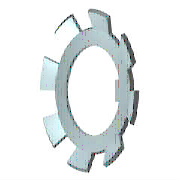
# Autodesk Inventor part: CSN 02 3640 - MB 33
Saved by Autodesk Inventor 2021 (Build 250183000, 183)
## iProperties
Created: 2020-01-21
Part Number: CSN 02 3640 - MB 33
Material: Steel, Mild
Description: Rolling bearings. Circular slotted nuts fo adapter and withdrawal sleeves
Document SubType Name: Modeling
Standard: CSN 02 3640
Designer: Angelos
Standards Organization: CSN
Language: en-US
Size Designation: MB 33
Categories: <MemberInstance><Categories><Category DisplayName="Shaft Parts" InternalName="7f7aeb1f-a693-4053-b835-cee3144e0d98" Mnemonic="SHFT"><Category DisplayName="Thrust Washers" InternalName="196297a3-bbf2-4c62-a426-6f1b43e49a92" Mnemonic="STWRDBRCMP"><CategoryParameter DisplayName="Diameter of Contact Area" InternalName="2e92645a-023d-4b6f-85cb-aa6579b07711" Mnemonic="conarea"/><CategoryParameter DisplayName="Groove Height" InternalName="459e1daf-c3a8-40cb-aa85-2a4675385d1b" Mnemonic="grvheig"/><CategoryParameter DisplayName="Thickness" InternalName="5f8ad5cd-5310-44ac-8ee3-8a10cbe3cc2a" Mnemonic="thick"/><CategoryParameter DisplayName="Shaft Diameter" InternalName="a5cdae98-95ea-47ec-9880-d704d388e74c" Mnemonic="shaftdia"/></Category></Category><Category DisplayName="DataType" InternalName="23b78d0f-2648-40c6-8793-ca6db495c9e8" Mnemonic="DATATYPE"><CategoryParameter DisplayName="DisplayName" InternalName="05415f3d-3907-474b-a020-eb9d644f4cf3" Mnemonic="DISPLAYNAME"/><CategoryParameter DisplayName="Standard" InternalName="0c0a119c-1e12-4c84-803f-101930972f5e" Mnemonic="STANDARD"/><CategoryParameter DisplayName="Description" InternalName="13903e3d-64b1-4950-80da-f627842ea37f" Mnemonic="DESCRIPTION"/><CategoryParameter DisplayName="Designation" InternalName="2675968c-4ce5-49e0-a4f5-552d29089031" Mnemonic="DESIGNATION"/><CategoryParameter DisplayName="Default Row" InternalName="2af9ec52-faaa-4026-b378-f9fa4afca842" Mnemonic="DEFAULTROW"/><CategoryParameter DisplayName="Folder Name" InternalName="3f06958e-8713-4116-9be7-ed6184ecc97b" Mnemonic="FOLDERNAME"/><CategoryParameter DisplayName="Revision Guid" InternalName="45a75005-10b1-4dfc-8d6d-dfe629f0b93c" Mnemonic="REVISIONGUID"/><CategoryParameter DisplayName="FileName" InternalName="8b46a4cc-9585-4fed-90c3-899f57e09a73" Mnemonic="FILENAME"/><CategoryParameter DisplayName="StdsOrg" InternalName="8f5914e1-4693-403f-8ab5-d37768198c9d" Mnemonic="STDSORG"/><CategoryParameter DisplayName="Family Version" InternalName="914462f6-6e19-4b14-ba84-155b9680b1d0" Mnemonic="FAMILYREVISION"/><CategoryParameter DisplayName="Standard Revision" InternalName="91d5a463-65c2-4fde-b823-3b7fea5e8e17" Mnemonic="STANDARDREVISION"/><CategoryParameter DisplayName="Member Revision" InternalName="a65d44b9-392f-4f4f-857b-e4b3d54996fe" Mnemonic="MEMBERREVISION"/><CategoryParameter DisplayName="ClipFormat" InternalName="bc51e27b-3422-4e78-93ef-cec197ddf230" Mnemonic="CLIPFORMAT"/><CategoryParameter DisplayName="Manufacturer" InternalName="cd6c7a72-a28a-4e50-99a9-2c7f4e13e5ad" Mnemonic="MANUFACTURER"/><CategoryParameter DisplayName="InternalName" InternalName="cf1d0246-76d9-4b4a-8305-fa0409afb5c1" Mnemonic="INTERNALNAME"/><CategoryParameter DisplayName="IsMetric" InternalName="e2385c5b-1ea4-4823-96a8-8de651266ec3" Mnemonic="ISMETRIC"/><Category DisplayName="Part" InternalName="c0e0b642-3bcb-4cc8-9e80-f96d35c4afa4" Mnemonic="PART"><CategoryParameter DisplayName="Part Number" InternalName="016b6077-bfbe-49bd-92c9-d8d59c39c941" Mnemonic="PARTNUMBER"/><CategoryParameter DisplayName="Stock Number" InternalName="4dba7c1c-e26c-444e-836c-b08b433409a8" Mnemonic="STOCKNUMBER"/><CategoryParameter DisplayName="Material Key" InternalName="5c9a8adb-dd2b-4535-b97f-0a94a95fe41f" Mnemonic="MATERIALKEY"/><CategoryParameter DisplayName="Material" InternalName="818a152a-d3c3-49ca-80ee-df7d91421b8e" Mnemonic="MATERIAL"/></Category></Category><Category DisplayName="LegacyMap" InternalName="cd87c42b-3e48-431e-b5c0-1cbeb14dfe77" Mnemonic="LEGACYMAP"><CategoryParameter DisplayName="unique DA member ID" InternalName="0918ad47-427f-4fed-ae26-24c81c58f590" Mnemonic="DACOOKIE"/><CategoryParameter DisplayName="Merge11 ID" InternalName="0ee8fb18-e2ed-4f39-96f6-1f4b5f50aa71" Mnemonic="MERGE11"/><CategoryParameter DisplayName="unique CC member ID" InternalName="5193edd4-b2b0-4ab4-9d54-de900eee34e0" Mnemonic="CCCOOKIE"/><CategoryParameter DisplayName="Split ID" InternalName="72b5c83c-be7f-45c4-ae51-9160ea6deb26" Mnemonic="SPLIT"/><CategoryParameter DisplayName="MemberID" InternalName="8e5e0294-fc51-4c8f-b3d7-003dc5ed94f6" Mnemonic="MEMBERID"/><CategoryParameter DisplayName="CatalogName" InternalName="d99d1e27-aa94-4de2-af4c-c348882a6f4f" Mnemonic="CATALOGNAME"/><CategoryParameter DisplayName="FamilyNumber" InternalName="e705e1f4-09cb-413e-91f9-551b4188271e" Mnemonic="FAMILYNUMBER"/></Category></Categories><FamilyTemplate Id="si0159"><FamilyTemplateParameters><FamilyTemplateParameter ObjectType="kUserParameterObject" ValueType="xs:double" Id="1" ObjectReferenceKey="TL"/><FamilyTemplateParameter ObjectType="kUserParameterObject" ValueType="xs:double" Id="2" ObjectReferenceKey="SD"/><FamilyTemplateParameter ObjectType="kUserParameterObject" ValueType="xs:double" Id="3" ObjectReferenceKey="RR"/><FamilyTemplateParameter ObjectType="kUserParameterObject" ValueType="xs:double" Id="4" ObjectReferenceKey="NND"/><FamilyTemplateParameter ObjectType="kUserParameterObject" ValueType="xs:double" Id="5" ObjectReferenceKey="SAZ"/><FamilyTemplateParameter ObjectType="kUserParameterObject" ValueType="xs:double" Id="6" ObjectReferenceKey="FAWI"/><FamilyTemplateParameter ObjectType="kUserParameterObject" ValueType="xs:double" Id="7" ObjectReferenceKey="PB"/><FamilyTemplateParameter ObjectType="kUserParameterObject" ValueType="xs:double" Id="8" ObjectReferenceKey="TW0"/><FamilyTemplateParameter ObjectType="kUserParameterObject" ValueType="xs:double" Id="9" ObjectReferenceKey="LADI"/><FamilyTemplateParameter ObjectType="kUserParameterObject" ValueType="xs:double" Id="10" ObjectReferenceKey="PNT"/><FamilyTemplateParameter ObjectType="kUserParameterObject" ValueType="xs:double" Id="11" ObjectReferenceKey="SD1"/><FamilyTemplateParameter ObjectType="kUserParameterObject" ValueType="xs:double" Id="12" ObjectReferenceKey="SD2"/><FamilyTemplateParameter ObjectType="kPropertyObject" ValueType="xs:string" Id="100" ObjectReferenceKey="{32853F0F-3444-11d1-9E93-0060B03C1CA6}" SubObjectId="52"/><FamilyTemplateParameter ObjectType="kPropertyObject" ValueType="xs:string" Id="105" ObjectReferenceKey="{32853F0F-3444-11d1-9E93-0060B03C1CA6}" SubObjectId="5"/><FamilyTemplateParameter ObjectType="kPartComponentDefinitionObject" ValueType="xs:string" Id="110" SubObjectId="Material"/></FamilyTemplateParameters></FamilyTemplate><CategoryParameterMap><ParamToTemplateMap><ParamToTemplate CategoryParameter="//CategoryParameter[@InternalName='05415f3d-3907-474b-a020-eb9d644f4cf3']" ConstantValue="CSN 02 3640"/><ParamToTemplate CategoryParameter="//CategoryParameter[@InternalName='cf1d0246-76d9-4b4a-8305-fa0409afb5c1']" ConstantValue="aa060291-c8e1-4752-be80-e0bdbd1a3c18"/><ParamToTemplate CategoryParameter="//CategoryParameter[@InternalName='3f06958e-8713-4116-9be7-ed6184ecc97b']" ConstantValue="CSN 02 3640 (2)"/><ParamToTemplate CategoryParameter="//CategoryParameter[@InternalName='914462f6-6e19-4b14-ba84-155b9680b1d0']" ConstantValue="10"/><ParamToTemplate CategoryParameter="//CategoryParameter[@InternalName='bc51e27b-3422-4e78-93ef-cec197ddf230']" ConstantValue="CF_INVENTOR.STDPARTS"/><ParamToTemplate CategoryParameter="//CategoryParameter[@InternalName='e2385c5b-1ea4-4823-96a8-8de651266ec3']" ConstantValue="true"/><ParamToTemplate CategoryParameter="//CategoryParameter[@InternalName='13903e3d-64b1-4950-80da-f627842ea37f']" ConstantValue="Rolling bearings. Circular slotted nuts fo adapter and withdrawal sleeves"/><ParamToTemplate CategoryParameter="//CategoryParameter[@InternalName='8f5914e1-4693-403f-8ab5-d37768198c9d']" ConstantValue="CSN"/><ParamToTemplate CategoryParameter="//CategoryParameter[@InternalName='0c0a119c-1e12-4c84-803f-101930972f5e']" ConstantValue="CSN 02 3640"/><ParamToTemplate CategoryParameter="//CategoryParameter[@InternalName='cd6c7a72-a28a-4e50-99a9-2c7f4e13e5ad']" TemplateParameter="104"/><ParamToTemplate CategoryParameter="//CategoryParameter[@InternalName='91d5a463-65c2-4fde-b823-3b7fea5e8e17']" TemplateParameter="103"/><ParamToTemplate CategoryParameter="//CategoryParameter[@InternalName='45a75005-10b1-4dfc-8d6d-dfe629f0b93c']" ConstantValue="53750fea-1528-4712-accf-1f7a3b85f0f9"/><ParamToTemplate CategoryParameter="//CategoryParameter[@InternalName='2af9ec52-faaa-4026-b378-f9fa4afca842']" ConstantValue="1"/><ParamToTemplate CategoryParameter="//CategoryParameter[@InternalName='d99d1e27-aa94-4de2-af4c-c348882a6f4f']" ConstantValue="CSN"/><ParamToTemplate CategoryParameter="//CategoryParameter[@InternalName='e705e1f4-09cb-413e-91f9-551b4188271e']" ConstantValue="145"/><ParamToTemplate CategoryParameter="//CategoryParameter[@InternalName='8b46a4cc-9585-4fed-90c3-899f57e09a73']" ConstantValue="CSN 02 3640 - MB 33"/><ParamToTemplate CategoryParameter="//CategoryParameter[@InternalName='a65d44b9-392f-4f4f-857b-e4b3d54996fe']" ConstantValue="8511a74e-8ed5-482c-baa0-05e7786f5d5e"/><ParamToTemplate CategoryParameter="//CategoryParameter[@InternalName='8e5e0294-fc51-4c8f-b3d7-003dc5ed94f6']" ConstantValue="39"/><ParamToTemplate CategoryParameter="//CategoryParameter[@InternalName='2675968c-4ce5-49e0-a4f5-552d29089031']" TemplateParameter="100"/><ParamToTemplate CategoryParameter="//CategoryParameter[@InternalName='818a152a-d3c3-49ca-80ee-df7d91421b8e']" TemplateParameter="110"/><ParamToTemplate CategoryParameter="//CategoryParameter[@InternalName='a5cdae98-95ea-47ec-9880-d704d388e74c']" TemplateParameter="4"/><ParamToTemplate CategoryParameter="//CategoryParameter[@InternalName='016b6077-bfbe-49bd-92c9-d8d59c39c941']" TemplateParameter="105"/><ParamToTemplate CategoryParameter="//CategoryParameter[@InternalName='5f8ad5cd-5310-44ac-8ee3-8a10cbe3cc2a']" TemplateParameter="2"/></ParamToTemplateMap></CategoryParameterMap></MemberInstance>
Density: 7.85 g/cm^3
Appearance: Semi-Polished
IsCustomPart: 0
Author: Angelos
Autodesk Inventor part; units mm, degrees
ref_plane "YZ Plane" through (0, 0, 0) normal (1, 0, 0) x (0, 1, 0)
ref_plane "XZ Plane" through (0, 0, 0) normal (0, 1, 0) x (-1, 0, 0)
sketch "Sketch1" plane through (0, 0, 0) normal (0, 0, 1) x (1, 0, 0)
  line L0 (-0.575278, 0) -> (3.451666, 0)
  line L1 (0, 3.9) -> (0, 11.6)
  line L2 (0, 97.054237) -> (6.503016, 111)
  line L3 (6.503016, 111) -> (8.768786, 109.943454)
  line L4 (8.768786, 109.943454) -> (2.5, 96.5)
  line L5 (2.5, 96.5) -> (2.5, 82.5)
  line L6 (2.5, 82.5) -> (0, 82.5)
  dimension "d1" = 2.5
  dimension "d2" = 165
  dimension "d3" = 193
  dimension "d4" = 222
  dimension "d5" = 25
  dimension "d6" = 2.5
  constraints: 10 end point, 3 perpendicular, 2 point on line, 1 parallel
  measures "d1" distance between parallel lines of L4 L2
  measures "d2" diameter of L6 L0
  measures "d3" diameter of L4.end L0
  measures "d4" diameter of L2.end L0
  measures "d5" angle of L1 L2
  measures "d6" distance between parallel lines of L1 L5
sketch "Sketch1 outline for Body" plane through (0, 0, 0) normal (0, 0, 1) x (1, 0, 0)
  line L0 (6.503016, 111) -> (0, 97.054237)
  line L1 (8.768786, 109.943454) -> (6.503016, 111)
  line L2 (2.5, 96.5) -> (8.768786, 109.943454)
  line L3 (2.5, 82.5) -> (2.5, 96.5)
  line L4 (0, 82.5) -> (2.5, 82.5)
  line L5 (0, 97.054237) -> (0, 82.5)
revolve "Body" add sketch "Sketch1 outline for Body" angle 360 about axis through (-10, 0, 0) along (1, 0, 0)
sketch "Sketch2" plane through (0, 0, 0) normal (-1, 0, 0) x (0, 0, 1)
  line L0 (0, -155.4) -> (0, 155.4)
  line L1 (9, 82.007622) -> (9, 75)
  line L2 (9, 75) -> (0, 75)
  line L3 (-9, 82.007622) -> (-9, 75)
  line L4 (-9, 75) -> (0, 75)
  line L5 (-155.4, 0) -> (155.4, 0)
  circle A0 centre (0, 0) radius 82.5
  circle A1 centre (0, 0) radius 111
  circle A2 centre (0, 0) radius 96.5
  line L6 (-7.968907, -96.170404) -> (-9.166307, -110.620879)
  line L7 (7.968907, -96.170404) -> (9.166307, -110.620879)
  line L8 (-7.968907, -96.170404) -> (0, 0) construction
  dimension "d9" = 18
  dimension "d10" = 75
  dimension "d16" = 4.73684
  constraints: 14 end point, 6 point on circle, 1 collinear, 1 parallel, 1 perpendicular, 1 point on line, 1 symmetric about line, 3 other
  measures "d9" diameter of L1 L0
  measures "d10" distance from line of L5 L2.end
  measures "d16" angle of L0 L6
extrude "Cut" cut sketch "Sketch2" against normal through all contours A1 L6 A2 L0 | L0 A2 L7 A1
extrude "Nib" add sketch "Sketch2" against normal blind 2.5 contours L4 L3 A0 L0 | L0 A0 L1 L2
pattern_circular "Cuts" count 19 over 360 about axis through (-10, 0, 0) along (1, 0, 0) of "Cut"
ref_plane "Work Plane1" through (1.25, 0, 0) normal (0, 0, -1) x (1, 0, 0)
equation "\"d1\" = SD"
equation "\"d2\" = SD1"
equation "\"d3\" = LADI"
equation "\"d4\" = SD2"
equation "\"d5\" = FAWI"
equation "\"d6\" = SD"
equation "\"d9\" = TW0"
equation "\"d10\" = 0.5 * SD1 - TL"
equation "\"d17\" = SD"
equation "\"d19\" = SD"
equation "\"FAWI\" = 25deg"
equation "\"SD1\" = NND"
equation "\"SD2\" = 222"
equation "\"SD\" = 2.5"
equation "\"TW0\" = PB"
equation "\"TL\" = PNT"
equation "\"LADI\" = 193"
equation "\"d8\" = SD1"
equation "\"RR\" = 0.1"
equation "\"NND\" = 165"
equation "\"PB\" = 18"
equation "\"PNT\" = 7.5"
body "Solid1"
